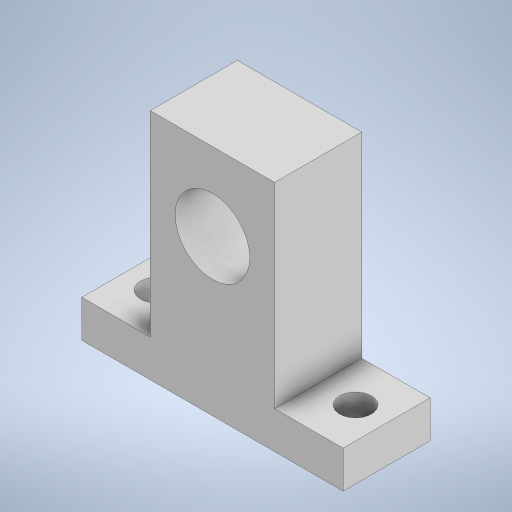
# Autodesk Inventor part: linear rod support mount
Saved by Autodesk Inventor 2023.2 (Build 272271000, 271)
## iProperties
Created: 2023-03-17
Part Number: linear rod support mount
Material: Generic
Document SubType Name: Modeling
Designer: dmargari
Density: 1 g/cm^3
Appearance: Default
Author: dmargari
Autodesk Inventor part; units mm, degrees
ref_plane "YZ Plane" through (0, 0, 0) normal (1, 0, 0) x (0, 1, 0)
ref_plane "XZ Plane" through (0, 0, 0) normal (0, 1, 0) x (-1, 0, 0)
ref_plane "XY Plane" through (0, 0, 0) normal (0, 0, 1) x (1, 0, 0)
sketch "Sketch1" plane through (0, 0, 0) normal (0, 0, 1) x (1, 0, 0)
  line L0 (10.9243, 48.5679) -> (30.9243, 48.5679)
  line L1 (30.9243, 48.5679) -> (30.9243, 17.0679)
  line L2 (30.9243, 17.0679) -> (10.9243, 17.0679)
  line L3 (10.9243, 17.0679) -> (10.9243, 48.5679)
  line L4 (10.9243, 48.5679) -> (30.9243, 17.0679) construction
  line L5 (30.9243, 48.5679) -> (10.9243, 17.0679) construction
  line L6 (-0.0757, 17.0679) -> (41.9243, 17.0679)
  line L7 (41.9243, 17.0679) -> (41.9243, 11.0679)
  line L8 (41.9243, 11.0679) -> (-0.0757, 11.0679)
  line L9 (-0.0757, 11.0679) -> (-0.0757, 17.0679)
  circle A0 centre (20.9243, 36.0679) radius 6
  point P0 (0, 0)
  point P1 (20.9243, 32.8179)
  point P2 (41.9243, 14.0679)
  point P3 (-0.0757, 14.0679)
  dimension "d0" = 20
  dimension "d1" = 31.5
  dimension "d2" = 6
  dimension "d3" = 42
  dimension "d4" = 11
  dimension "d5" = 12
  dimension "d6" = 25
  constraints: 20 end point, 4 midpoint, 4 perpendicular, 2 parallel, 2 point on line, 1 centre point, 1 horizontal
  measures "d0" distance of L1.end L2.end
  measures "d1" distance of L0.end L1.end
  measures "d2" distance between parallel lines of L6 L8
  measures "d3" distance of point (41.924, 14.068) point (-0.076, 14.068)
  measures "d4" distance between parallel lines of L3 L9
  measures "d5" diameter of A0
  measures "d6" distance from line of L8 A0.centre
extrude "Extrusion1" add sketch "Sketch1" along normal mid plane 14
sketch "Sketch2" plane through (-0.0757, 11.0679, 7) normal (0, -1, 0) x (1, 0, 0)
  line L0 (42, -14) -> (42, 0) construction
  line L1 (42, -7) -> (0.0757, -7) construction
  line L2 (0, -14) -> (0, 0) projected
  point P0 (37, -7)
  point P1 (5, -7)
  point P2 (0, -7)
  dimension "d9" = 5
  dimension "d10" = 5
  constraints: 3 midpoint, 2 end point, 2 point on line, 1 horizontal
  measures "d9" distance of point (42, -7) point (37, -7)
  measures "d10" distance of point (0, -7) point (5, -7)
hole "Hole1" at (36.9243, 11.0679, 0) at (4.9243, 11.0679, 0) direction (0, 1, 0) diameter 5.1 end through all
body "Solid1"
